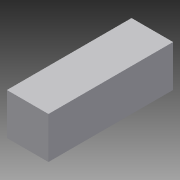
# Autodesk Inventor part: 4x4x12 PG-27 Machine Key
Saved by Autodesk Inventor 2013 (Build 170138000, 138)
## iProperties
Created: 2013-01-30
Part Number: 4x4x12 PG-27 Machine Key
Material: Generic
Document SubType Name: Modeling
Designer: carneeki
Density: 1 g/cm^3
Author: carneeki
Autodesk Inventor part; units mm, degrees
ref_plane "YZ Plane" through (0, 0, 0) normal (1, 0, 0) x (0, 1, 0)
ref_plane "XZ Plane" through (0, 0, 0) normal (0, 1, 0) x (-1, 0, 0)
ref_plane "XY Plane" through (0, 0, 0) normal (0, 0, 1) x (1, 0, 0)
sketch "Sketch1" plane through (0, 0, 0) normal (0, 0, 1) x (1, 0, 0)
  line L0 (-4.6136, -2) -> (-0.6136, -2)
  line L1 (-0.6136, -2) -> (-0.6136, 2)
  line L2 (-0.6136, 2) -> (-4.6136, 2)
  line L3 (-4.6136, 2) -> (-4.6136, -2)
  line L4 (-4.6136, -2) -> (-0.6136, 2) construction
  line L5 (-0.6136, -2) -> (-4.6136, 2) construction
  point P0 (0, 0)
  point P1 (-2.6136, 0)
  dimension "d0" = 4
  dimension "d1" = 4
  constraints: 12 end point, 2 midpoint, 2 parallel, 1 horizontal, 1 perpendicular
  measures "d0" distance of L2.end L1.end
  measures "d1" distance of L1.end L0.end
extrude "Extrusion1" add sketch "Sketch1" along normal blind 12
body "Solid1"
